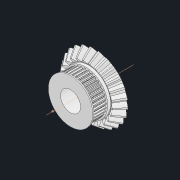
# Autodesk Inventor part: かさ歯車1
Saved by Autodesk Inventor 2021 (Build 250183000, 183)
## iProperties
CustomPartVersion: 1
Created: 2021-07-25
Part Number: かさ歯車1
Material: ABS プラスチック
Document SubType Name: Modeling
Designer: yuto6
Categories: <?xml version="1.0" encoding="UTF-16"?> <MemberInstance><Categories><FamilyTemplate><FamilyTemplateParameter ValueType="xs:double" Id="1" ObjectReferenceKey="da_z" ObjectType="kUserParameterObject"/><FamilyTemplateParameter ValueType="xs:double" Id="2" ObjectReferenceKey="da_b" ObjectType="kUserParameterObject"/><FamilyTemplateParameter ValueType="xs:double" Id="3" ObjectReferenceKey="da_beta" ObjectType="kUserParameterObject"/><FamilyTemplateParameter ValueType="xs:double" Id="4" ObjectReferenceKey="da_dae" ObjectType="kUserParameterObject"/><FamilyTemplateParameter ValueType="xs:double" Id="5" ObjectReferenceKey="da_ve" ObjectType="kUserParameterObject"/><FamilyTemplateParameter ValueType="xs:double" Id="6" ObjectReferenceKey="da_omega" ObjectType="kUserParameterObject"/><FamilyTemplateParameter ValueType="xs:string" Id="7" ObjectReferenceKey="EAIAABAAAAAAHwAAAAAAAIAAAAAAAAAA" ObjectType="83914240" SubObjectId="SurfaceGeometry"/></FamilyTemplate><ParamToTemplateMap><ParamToTemplate CategoryParameter="//CategoryParameter[@InternalName='046C89C9-8512-4d59-83FE-43B91F4F132A']" TemplateParameter="1"/><ParamToTemplate CategoryParameter="//CategoryParameter[@InternalName='2552DF32-E462-4b46-AEBF-C6C7768E72AC']" TemplateParameter="2"/><ParamToTemplate CategoryParameter="//CategoryParameter[@InternalName='C9EE641D-15FC-4fae-A226-E94C4372FDD7']" TemplateParameter="3"/><ParamToTemplate><ParamToTemplate CategoryParameter="//CategoryParameter[@InternalName='00B6519A-459B-49c7-AD84-2E56D39A5744']" ConstantValue="0.000000"/></ParamToTemplate><ParamToTemplate><ParamToTemplate CategoryParameter="//CategoryParameter[@InternalName='04B31F0E-C7A6-4894-AA32-9629BEFACF47']" ConstantValue="1.000000"/></ParamToTemplate><ParamToTemplate><ParamToTemplate CategoryParameter="//CategoryParameter[@InternalName='43CBEC2E-7847-49e7-A936-2F7889FCB2D9']" ConstantValue="0.200000"/></ParamToTemplate><ParamToTemplate><ParamToTemplate CategoryParameter="//CategoryParameter[@InternalName='B1EFC894-105D-4ebd-86BF-FA20ED196853']" ConstantValue="0.300000"/></ParamToTemplate><ParamToTemplate><ParamToTemplate CategoryParameter="//CategoryParameter[@InternalName='51175063-3D10-4879-93E8-6246FE8B403D']" ConstantValue="2060000000.000000"/></ParamToTemplate><ParamToTemplate><ParamToTemplate CategoryParameter="//CategoryParameter[@InternalName='A3A52E27-4454-46a9-B0BD-C932399B70AF']" ConstantValue="0.300000"/></ParamToTemplate><ParamToTemplate CategoryParameter="//CategoryParameter[@InternalName='2A200944-5A8C-41ca-B96E-8520D2E510F1']" TemplateParameter="4"/><ParamToTemplate><ParamToTemplate CategoryParameter="//CategoryParameter[@InternalName='1A637F62-92C8-44bc-B81F-10802510B579']" ConstantValue="4.211157"/></ParamToTemplate><ParamToTemplate CategoryParameter="//CategoryParameter[@InternalName='B52DD4BE-6863-48fb-BF58-89EF6F9EC65C']" TemplateParameter="5"/><ParamToTemplate><ParamToTemplate CategoryParameter="//CategoryParameter[@InternalName='3956BFF2-84D2-457d-93C2-9B0613DEBA67']" ConstantValue="2.675717"/></ParamToTemplate><ParamToTemplate CategoryParameter="//CategoryParameter[@InternalName='739CFA02-461B-4bf8-8049-181FCAD8B28F']" TemplateParameter="6"/><ParamToTemplate><ParamToTemplate CategoryParameter="//CategoryParameter[@InternalName='A27E999F-E2CE-4481-8A2A-EBF499C4C3C5']" ConstantValue="0.000000"/></ParamToTemplate><ParamToTemplate><ParamToTemplate CategoryParameter="//CategoryParameter[@InternalName='9E1B4470-B2D3-4ff1-B813-535BB4CDF51A']" ConstantValue="3520000.000000"/></ParamToTemplate><ParamToTemplate><ParamToTemplate CategoryParameter="//CategoryParameter[@InternalName='F8452263-BFF6-458c-9FB1-07C4B99E95CD']" ConstantValue="11400000.000000"/></ParamToTemplate><ParamToTemplate><ParamToTemplate CategoryParameter="//CategoryParameter[@InternalName='3E3BB259-FD49-497f-8171-6EBC954A3479']" ConstantValue="2.000000"/></ParamToTemplate><ParamToTemplate CategoryParameter="//CategoryParameter[@InternalName='27C3BAF2-7550-4e4b-AE2C-0DB134B7D9B7']" TemplateParameter="7"/></ParamToTemplateMap><Category DisplayName="Gear" InternalName="DC85795E-93AB-48d5-8EEE-5A27447B64BD" Mnemonic="Gear"><CategoryParameter DisplayName="z" InternalName="046C89C9-8512-4d59-83FE-43B91F4F132A" Mnemonic="z"/><CategoryParameter DisplayName="b" InternalName="2552DF32-E462-4b46-AEBF-C6C7768E72AC" Mnemonic="b"/><CategoryParameter DisplayName="||b|" InternalName="C9EE641D-15FC-4fae-A226-E94C4372FDD7" Mnemonic="beta"/><CategoryParameter DisplayName="x" InternalName="00B6519A-459B-49c7-AD84-2E56D39A5744" Mnemonic="x"/><CategoryParameter DisplayName="a*" InternalName="04B31F0E-C7A6-4894-AA32-9629BEFACF47" Mnemonic="a"/><CategoryParameter DisplayName="c*" InternalName="43CBEC2E-7847-49e7-A936-2F7889FCB2D9" Mnemonic="c"/><CategoryParameter DisplayName="r|.f|*" InternalName="B1EFC894-105D-4ebd-86BF-FA20ED196853" Mnemonic="rf"/><CategoryParameter DisplayName="E" InternalName="51175063-3D10-4879-93E8-6246FE8B403D" Mnemonic="E"/><CategoryParameter DisplayName="||m|" InternalName="A3A52E27-4454-46a9-B0BD-C932399B70AF" Mnemonic="mi"/><Category DisplayName="BevelGear" InternalName="0C98F69A-0C2B-4791-B2FE-7691BB227E77" Mnemonic="BevelGear"><CategoryParameter DisplayName="d|.ae|" InternalName="2A200944-5A8C-41ca-B96E-8520D2E510F1" Mnemonic="dae"/><CategoryParameter DisplayName="d|.ai|" InternalName="1A637F62-92C8-44bc-B81F-10802510B579" Mnemonic="dai"/><CategoryParameter DisplayName="J|.e|" InternalName="B52DD4BE-6863-48fb-BF58-89EF6F9EC65C" Mnemonic="ve"/><CategoryParameter DisplayName="J|.i|" InternalName="3956BFF2-84D2-457d-93C2-9B0613DEBA67" Mnemonic="vi"/><CategoryParameter DisplayName="||S|" InternalName="739CFA02-461B-4bf8-8049-181FCAD8B28F" Mnemonic="omega"/><CategoryParameter DisplayName="x|.t|" InternalName="A27E999F-E2CE-4481-8A2A-EBF499C4C3C5" Mnemonic="xt"/><CategoryParameter DisplayName="||s||.Flim|" InternalName="9E1B4470-B2D3-4ff1-B813-535BB4CDF51A" Mnemonic="sFlim"/><CategoryParameter DisplayName="||s||.Hlim|" InternalName="F8452263-BFF6-458c-9FB1-07C4B99E95CD" Mnemonic="sHlim"/><CategoryParameter DisplayName="種類" InternalName="3E3BB259-FD49-497f-8171-6EBC954A3479" Mnemonic="type"/><CategoryParameter DisplayName="PitchDiameter" InternalName="27C3BAF2-7550-4e4b-AE2C-0DB134B7D9B7" Mnemonic="IDS_PITCHDIAM"/></Category></Category></Categories></MemberInstance>
Mass: 22.094 g
Surface Area: 88.6811 cm^2
Volume: 20.8434 cm^3
Density: 1.06 g/cm^3
Appearance: 滑らか - 白
Author: yuto6
Autodesk Inventor part; units mm, degrees
ref_plane "メッシュ平面2" through (0, 0, 0) normal (0.9921147, 0.1253332, 0) x (0, 0, 1)
sketch "歯のボディ スケッチ" plane through (0, 0, 0) normal (1, 0, 0) x (0, 1, 0)
  line L0 (0, 0) -> (23.047, -36.395) construction
  line L1 (23.047, -36.395) -> (26.6275, -33.8375)
  line L2 (26.6275, -33.8375) -> (0, 0) construction
  line L3 (25, -35) -> (0, 0) construction
  line L4 (18.2245, -28.7795) -> (21.0558, -26.7572)
  line L5 (23.047, -36.395) -> (18.2245, -28.7795)
  line L6 (26.6275, -33.8375) -> (21.0558, -26.7572)
  line L7 (0, -44.8427) -> (0, 7.4738) projected
  line L8 (0, -35) -> (26.6275, -35) construction
  dimension "d0" = 50
  dimension "d1" = 46.0941
  dimension "d2" = 53.2549
  dimension "d3" = 9
  dimension "d4" = 33.8375
  constraints: 16 end point, 4 point on line, 3 perpendicular, 2 collinear, 1 horizontal alignment, 1 vertical alignment
  measures "d0" diameter of L3.start L7
  measures "d1" diameter of L0.end L7
  measures "d2" diameter of L1.end L7
  measures "d3" distance between parallel lines of L1 L4
  measures "d4" vertical distance of L1.end L0.start
revolve "歯のボディ" add sketch "歯のボディ スケッチ" angle 360 about axis through (0, 0, 0) along (0, 0, 1)
ref_plane "歯の平面" through (0, 25, -35) normal (0, -0.5812382, 0.8137335) x (1, 0, 0)
sketch "開始スケッチ" plane through (0, 25, -35) normal (0, -0.5812382, 0.8137335) x (1, 0, 0)
  line L0 (0, -37.1929) -> (0, 10.099) projected
  arc A0 (-0.7892, -2.928) -> (-3.6319, 3.1257) centre (-11.8767, -4.44) ccw
  arc A1 (3.6319, 3.1257) -> (0.7892, -2.928) centre (11.8767, -4.44) ccw
  line L1 (-0.7892, -2.928) -> (0.7892, -2.928)
  arc A2 (3.6319, 3.1257) -> (-3.6319, 3.1257) centre (0, -30.7226) ccw
  dimension "d7" = 11.19
  dimension "d8" = 11.8767
  dimension "d9" = 26.2826
  dimension "d57" = 34.0426
  dimension "d58" = 27.7946
  constraints: 6 point on circle, 3 centre point, 3 symmetric about line, 2 end point, 1 coincident, 1 perpendicular, 1 other
  measures "d7" radius of A0
  measures "d8" horizontal distance of point (0, -30.723) A0.centre
  measures "d9" vertical distance of point (0, -30.723) A0.centre
  measures "d57" radius of A2
  measures "d58" distance from line of A2.centre L1
ref_plane "終了側平面" through (0, 19.641, -27.4974) normal (0, -0.5812382, 0.8137335) x (1, 0, 0)
sketch "終了側スケッチ" plane through (0, 19.641, -27.4974) normal (0, -0.5812382, 0.8137335) x (1, 0, 0)
  line L0 (0, -29.369) -> (0, 7.9746) projected
  arc A0 (-0.6201, -2.3004) -> (-2.8533, 2.4557) centre (-9.3308, -3.4883) ccw
  arc A1 (2.8533, 2.4557) -> (0.6201, -2.3004) centre (9.3308, -3.4883) ccw
  line L1 (-0.6201, -2.3004) -> (0.6201, -2.3004)
  arc A2 (2.8533, 2.4557) -> (-2.8533, 2.4557) centre (0, -24.1369) ccw
  dimension "d12" = 8.7913
  dimension "d15" = 9.3308
  dimension "d16" = 20.6486
  dimension "d59" = 26.7452
  dimension "d60" = 21.8365
  constraints: 6 point on circle, 3 centre point, 3 symmetric about line, 2 end point, 1 coincident, 1 other
  measures "d12" radius of A0
  measures "d15" horizontal distance of A0.centre point (0, -24.137)
  measures "d16" vertical distance of A0.centre point (0, -24.137)
  measures "d59" radius of A2
  measures "d60" distance from line of A2.centre L1
loft "Loft" cut profiles "開始スケッチ", "終了側スケッチ"
pattern_circular "Circular Pattern" count 25 over 360 about axis through (0, 0, 0) along (0, 0, 1) of "Loft"
sketch3d "3D スケッチ(右)"
ref_plane "終了側平面(右)" through (-5.1328, 18.9584, -27.4974) normal (0.1518966, -0.5610394, 0.8137335) x (0.9652487, 0.2613328, 0)
sketch "終了側スケッチ(右)" plane through (-5.1328, 18.9584, -27.4974) normal (0.1518966, -0.5610394, 0.8137335) x (0.9652487, 0.2613328, 0)
  arc A0 (-0.6201, -2.3004) -> (-2.8533, 2.4557) centre (-9.3308, -3.4883) ccw
  line L0 (0, -34.8401) -> (0, 13.343) projected
  arc A1 (2.8533, 2.4557) -> (0.6201, -2.3004) centre (9.3308, -3.4883) ccw
  line L1 (-0.6201, -2.3004) -> (0.6201, -2.3004)
  arc A2 (2.8533, 2.4557) -> (-2.8533, 2.4557) centre (0, -24.1369) ccw
  dimension "d70" = 9.3308
  dimension "d71" = 20.6486
  dimension "d72" = 8.7913
  dimension "d73" = 21.8365
  dimension "d74" = 26.7452
  constraints: 6 point on circle, 3 centre point, 3 symmetric about line, 2 end point, 1 coincident, 1 perpendicular, 1 other
  measures "d70" horizontal distance of A2.centre A0.centre
  measures "d71" vertical distance of point (0, -24.137) A0.centre
  measures "d72" radius of A0
  measures "d73" distance from line of point (0, -24.137) L1
  measures "d74" radius of A2
feature "ロフト(右)" [suppressed]
pattern_circular "放射状パターン(右)" [suppressed]
sketch3d "3D スケッチ(左)"
ref_plane "終了側平面(左)" through (5.1706, 18.9584, -27.5234) normal (-0.1528933, -0.5605929, 0.8138546) x (0.9647619, -0.2631244, 0)
sketch "終了側スケッチ(左)" plane through (5.1706, 18.9584, -27.5234) normal (-0.1528933, -0.5605929, 0.8138546) x (0.9647619, -0.2631244, 0)
  line L0 (0, -52.6029) -> (0, 22.0608) projected
  arc A0 (-0.6201, -2.2933) -> (-2.8533, 2.4627) centre (-9.3308, -3.4812) ccw
  arc A1 (2.8533, 2.4627) -> (0.6201, -2.2933) centre (9.3308, -3.4812) ccw
  line L1 (-0.6201, -2.2933) -> (0.6201, -2.2933)
  ellipse E0 centre (0, -15.5477) end of major axis (21.0558, -15.5477) minor radius 17.1363 projected
  arc A2 (2.8533, 2.4627) -> (-2.8533, 2.4627) centre (0, -24.1298) ccw
  dimension "d56" = 17.1363
  dimension "d30" = 8.7913
  dimension "d31" = 9.3308
  dimension "d32" = 20.6486
  dimension "d61" = 26.7452
  dimension "d62" = 21.8365
  constraints: 6 point on circle, 3 centre point, 3 symmetric about line, 2 end point, 1 coincident, 2 other
  measures "d30" radius of A0
  measures "d31" horizontal distance of point (0, -24.13) A0.centre
  measures "d32" vertical distance of A0.centre point (0, -24.13)
  measures "d61" radius of A2
  measures "d62" distance from line of point (0, -24.13) L1
feature "ロフト(左)" [suppressed]
pattern_circular "放射状パターン(左)" [suppressed]
sketch "ボディ スケッチ" plane through (0, 0, 0) normal (1, 0, 0) x (0, 1, 0)
  line L0 (0, -38.9036) -> (0, -28.1608) projected
  line L1 (23.047, -36.395) -> (18.2245, -28.7795) projected
  line L2 (18.2245, -28.7795) -> (0, -28.7795)
  line L3 (23.047, -36.395) -> (0, -36.395)
  constraints: 4 end point, 2 perpendicular, 2 point on line
revolve "固定ボディ" add sketch "ボディ スケッチ" angle 360 about axis through (0, 0, 0) along (0, 0, 1)
sketch "Sketch6" plane through (0, 0, 0) normal (1, 0, 0) x (0, 1, 0)
  line L0 (25, -35) -> (0, 0) projected
  line L1 (0, -43.2) -> (0, 7.2) projected
surface revolve "ピッチ円直径" sketch "Sketch6" angle 360 about axis through (0, 0, 0) along (0, 0, 1) shown no curves L0
ref_plane "作業平面6" through (0, 0, -26.35) normal (0, 0, -1) x (-0.5877853, -0.809017, 0)
sketch "スケッチ10" plane through (0, 0, -26.35) normal (0, 0, -1) x (-0.5877853, -0.809017, 0)
  circle A0 centre (0, 0) radius 17.8075
  dimension "d143" = 35.615
  constraints: 1 centre point, 1 coincident
  measures "d143" diameter of A0
extrude "押し出し1" add sketch "スケッチ10" along normal up to next
sketch "スケッチ14" plane through (0, 0, -26.35) normal (0, 0, 1) x (1, 0, 0)
  circle A0 centre (0, 0) radius 17.1887 construction
  circle A1 centre (0, 0) radius 16.8077
  circle A2 centre (0, 0) radius 15.6977
  line L0 (17.1887, 0) -> (17.0781, -1.9469) construction
  circle A3 centre (17.0781, -1.9469) radius 1.975
  circle A4 centre (17.1887, 0) radius 1.975
  point P0 (0, 16.8077)
  point P1 (15.6489, -1.2368)
  point P2 (16.6985, -1.9132)
  point P3 (16.8077, 0.0095)
  point P4 (15.6883, -0.5436)
  dimension "d144" = 34.3775
  dimension "d145" = 0.381
  dimension "d146" = 1.11
  dimension "d147" = 3.95
  dimension "d148" = 1.95
  dimension "d149" = 3.95
  constraints: 4 centre point, 4 coincident, 2 end point, 2 point on circle, 1 horizontal alignment, 1 vertical alignment, 3 other
  measures "d144" diameter of A0
  measures "d147" diameter of A3
  measures "d148" distance of L0.start L0.end
  measures "d149" diameter of A4
extrude "押し出し2" add sketch "スケッチ14" along normal blind 11 contours A1 A4 A2 A3 | A3 A2 A4 A1 | A1 A3 A2 A4 | A4 A2 A3 A1 | A3 A4 A2 | A2 A4 A3 | A2 A3 A4 | A4 A3 A2
extrude "押し出し3" cut sketch "スケッチ14" along normal through all contours A1 A4 A2 A3 picked at (16.4067, -0.974)
fillet "フィレット2" radius 0.15 2 edges at (15.6489, -1.2368, -20.85) (15.6883, -0.5436, -20.85)
fillet "フィレット3" radius 0.285 2 edges at (16.6985, -1.9132, -20.85) (16.8077, 0.0095, -20.85)
pattern_circular "円形状パターン4" count 36 over 360 about axis through (0, 0, 0) along (0, 0, 1) of "押し出し3", "フィレット2", "フィレット3"
sketch "スケッチ15" plane through (0, 0, -15.35) normal (0, 0, 1) x (1, 0, 0)
  circle A0 centre (0, 0) radius 17.8075 projected
extrude "押し出し4" add sketch "スケッチ15" along normal blind 1
sketch "スケッチ18" plane through (0, 0, -14.35) normal (0, 0, 1) x (1, 0, 0)
  circle A0 centre (0, 0) radius 8
  dimension "d165" = 16
  constraints: 1 centre point, 1 coincident
  measures "d165" diameter of A0
extrude "押し出し6" cut sketch "スケッチ18" against normal through all
equation "\"d0\" = da_de"
equation "\"d1\" = da_dfe"
equation "\"d2\" = da_dae"
equation "\"d3\" = da_b"
equation "\"d4\" = da_ve"
equation "\"d7\" = fd_rr"
equation "\"d8\" = fd_x"
equation "\"d9\" = fd_y"
equation "\"d57\" = 0.5 * fd_dva + 0.3 * da_he"
equation "\"d58\" = 0.5 * fd_dva - 1.12 * da_he"
equation "\"da_teethtype\" = 0"
equation "\"d149\" = d147"
equation "\"da_b\" = 9"
equation "\"da_de\" = 50"
equation "\"da_dae\" = 53.25493"
equation "\"da_dfe\" = 46.09408"
equation "\"da_le\" = 43.01163"
equation "\"da_omega\" = 90deg"
equation "\"da_beta\" = 0"
equation "\"da_delta\" = 35.537678deg"
equation "\"da_alpha\" = 20deg"
equation "\"da_he\" = 4.4"
equation "\"da_ve\" = 33.83752"
equation "\"da_zv\" = 30.72259"
equation "\"fd_loft\" = da_b + 0.05 * da_he"
equation "\"fd_x\" = fd_x1 + fd_x2"
equation "\"fd_y\" = fd_y1 - fd_y2"
equation "\"fd_dd\" = fd_dva - 0.8 * da_he"
equation "\"da_dvw\" = 61.44518"
equation "\"d11\" = fd_loft"
equation "\"da_dm\" = 44.76886"
equation "\"da_x\" = 0"
equation "\"da_m\" = 2"
equation "\"d50\" = da_omega"
equation "\"fd_rr\" = 11.190047"
equation "\"fd_dva\" = 65.44518"
equation "\"fd_x1\" = 1.587542"
equation "\"fd_x2\" = 10.289124"
equation "\"fd_y1\" = 30.681546"
equation "\"fd_y2\" = 4.398985"
body "Solid1"
body "Srf1"
